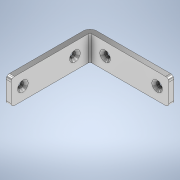
# Autodesk Inventor part: Right Bracket 50mm RS749-1680
Saved by Autodesk Inventor 2021 (Build 250183000, 183)
## iProperties
Created: 2020-07-14
Part Number: Right Bracket 50mm RS749-1680
Material: Stainless Steel
Document SubType Name: Modeling
Designer: jgray
Density: 8 g/cm^3
Appearance: Steel - Polished
Author: jgray
Autodesk Inventor part; units mm, degrees
ref_plane "YZ Plane" through (0, 0, 0) normal (1, 0, 0) x (0, 1, 0)
ref_plane "XZ Plane" through (0, 0, 0) normal (0, 1, 0) x (-1, 0, 0)
ref_plane "XY Plane" through (0, 0, 0) normal (0, 0, 1) x (1, 0, 0)
sketch "Sketch1" plane through (0, 0, 0) normal (0, 1, 0) x (-1, 0, 0)
  line L0 (0, 0) -> (50, 0)
  line L1 (50, 0) -> (50, -46)
  line L2 (46, -50) -> (0, -50)
  line L3 (0, -50) -> (0, 0)
  arc A0 (46, -50) -> (50, -46) centre (46, -46) ccw
  line L4 (0, 0) -> (47, 0)
  line L5 (47, 0) -> (47, -46)
  line L6 (46, -47) -> (0, -47)
  line L7 (0, -47) -> (0, 0)
  arc A1 (46, -47) -> (47, -46) centre (46, -46) ccw
  point P0 (50, -50)
  point P1 (47, -47)
  dimension "d0" = 50
  dimension "d1" = 50
  dimension "d2" = 4
  dimension "d3" = 47
  dimension "d4" = 47
  dimension "d5" = 1
  constraints: 16 end point, 4 parallel, 4 point on circle, 4 point on line, 4 tangent, 2 centre point, 2 horizontal, 2 perpendicular
  measures "d0" distance of point (50, -50) L2.end
  measures "d1" distance of L0.end point (50, -50)
  measures "d2" radius of A0
  measures "d3" distance of point (47, -47) L6.end
  measures "d4" distance of L4.end point (47, -47)
  measures "d5" radius of A1
extrude "Extrusion1" add sketch "Sketch1" along normal blind 15 contours L0 L1 A0 L2 L3 L6 A1 L5
fillet "Fillet1" radius 2 4 edges at (-48.5, 15, 0) (-48.5, 0, 0) (0, 15, -48.5) (0, 0, -48.5)
sketch "Sketch2" plane through (-47, 0, -46) normal (1, 0, 0) x (0, 0, -1)
  line L0 (-57.4618, 7.5) -> (28.1267, 7.5) construction
  line L1 (-46, 2) -> (-46, 13) projected
  point P0 (-46, 0)
  point P1 (-46, 7.5)
  point P2 (-39, 7.5)
  point P3 (-8, 7.5)
  dimension "d9" = 7
  dimension "d10" = 31
  constraints: 3 point on line, 2 end point, 1 horizontal, 1 midpoint
  measures "d9" distance from line of L1 point (-39, 7.5)
  measures "d10" distance of point (-8, 7.5) point (-39, 7.5)
hole "Hole1" at (-47, 7.5, -7) at (-47, 7.5, -38) direction (-1, 0, 0) diameter 3.5 end through all countersink diameter 6.3 countersink angle 90 clearance for "Countersunk Flat Head Screw ISO 2009/7046" size "M3" standard "ISO"
sketch "Sketch3" plane through (-46, 0, -47) normal (0, 0, 1) x (1, 0, 0)
  line L0 (63.5676, 7.5) -> (-29.6264, 7.5) construction
  line L1 (46, 2) -> (46, 13) construction
  arc A0 (44, 0) -> (46, 2) centre (44, 2) ccw projected
  line L2 (46, 2) -> (46, 13) projected
  arc A1 (46, 13) -> (44, 15) centre (44, 13) ccw projected
  line L3 (0, 15) -> (44, 15) projected
  line L4 (0, 0) -> (0, 15) projected
  line L5 (0, 0) -> (44, 0) projected
  point P0 (46, 0)
  point P1 (46, 7.5)
  point P2 (39, 7.5)
  point P3 (8, 7.5)
  dimension "d18" = 7
  dimension "d19" = 31
  constraints: 3 point on line, 2 end point, 1 horizontal, 1 midpoint
  measures "d18" distance from line of point (39, 7.5) L1
  measures "d19" distance of point (8, 7.5) point (39, 7.5)
hole "Hole2" at (-7, 7.5, -47) at (-38, 7.5, -47) direction (0, 0, -1) diameter 3.5 end through all countersink diameter 6.3 countersink angle 90 clearance for "Countersunk Flat Head Screw ISO 2009/7046" size "M3" standard "ISO"
body "Solid1"
